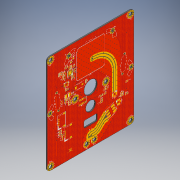
# Autodesk Inventor part: +XPanel_PCB
Saved by Autodesk Inventor 2018 (Build 220112000, 112)
## iProperties
Created: 2018-10-25
Part Number: +XPanel_PCB
Material: Epoxy Resin
Document SubType Name: Modeling
Designer: Bradley
Density: 1.14 g/cm^3
Appearance: Smooth - Dark Gray
Author: Bradley
Autodesk Inventor part; units mm, degrees
ref_plane "YZ Plane" through (0, 0, 0) normal (1, 0, 0) x (0, 1, 0)
ref_plane "XZ Plane" through (0, 0, 0) normal (0, 1, 0) x (-1, 0, 0)
ref_plane "XY Plane" through (0, 0, 0) normal (0, 0, 1) x (1, 0, 0)
sketch "Sketch1" plane through (0, 0, 0) normal (1, 0, 0) x (0, 1, 0)
  line L0 (36.5, -42) -> (-36.5, -42) construction
  line L1 (-36.5, -42) -> (-36.5, 42) construction
  line L2 (-36.5, 42) -> (36.5, 42) construction
  line L3 (36.5, 42) -> (36.5, -42) construction
  line L4 (36.5, -42) -> (-36.5, 42) construction
  line L5 (-36.5, -42) -> (36.5, 42) construction
  line L6 (-14, 0) -> (14, 0) construction
  line L7 (-39.5, -42) -> (-39.5, 42)
  arc A0 (-36.5, 45) -> (-39.5, 42) centre (-36.5, 42) ccw
  line L8 (-36.5, 45) -> (36.5, 45)
  arc A1 (39.5, 42) -> (36.5, 45) centre (36.5, 42) ccw
  line L9 (39.5, 42) -> (39.5, -42)
  arc A2 (36.5, -45) -> (39.5, -42) centre (36.5, -42) ccw
  line L10 (36.5, -45) -> (-36.5, -45)
  arc A3 (-39.5, -42) -> (-36.5, -45) centre (-36.5, -42) ccw
  point P0 (0, 0)
  point P1 (0, 0)
  dimension "d2" = 28
  dimension "d3" = 79
  dimension "d117" = 3
  dimension "d118" = 90
  dimension "d119" = 84
  dimension "d120" = 73
  constraints: 22 end point, 8 point on circle, 6 tangent, 4 centre point, 4 coincident, 4 midpoint, 4 parallel, 2 horizontal, 2 perpendicular, 1 equal radius, 1 vertical
  measures "d2" distance of L6.start L6.end
  measures "d3" distance between parallel lines of L9 L7
  measures "d117" radius of A0
  measures "d118" distance between parallel lines of L10 L8
  measures "d119" distance of L0.end L1.end
  measures "d120" distance of L1.end L2.end
extrude "Extrusion1" add sketch "Sketch1" along normal mid plane 1
sketch "Sketch3" plane through (0.5, 0, 0) normal (1, 0, 0) x (0, 0, -1)
  circle A0 centre (-2.5, 0) radius 6
  circle A1 centre (12.35, 0) radius 4.5
  line L0 (26, -6) -> (22, -6)
  line L1 (21, -5) -> (21, 5)
  line L2 (22, 6) -> (26, 6)
  line L3 (27, 5) -> (27, -5)
  line L4 (27, -6) -> (21, 6) construction
  line L5 (21, -6) -> (27, 6) construction
  arc A2 (21, -5) -> (22, -6) centre (22, -5) ccw
  arc A3 (26, -6) -> (27, -5) centre (26, -5) ccw
  arc A4 (27, 5) -> (26, 6) centre (26, 5) ccw
  arc A5 (22, 6) -> (21, 5) centre (22, 5) ccw
  point P0 (0, 0)
  point P1 (24, 0)
  point P2 (24, 0)
  dimension "d15" = 2.5
  dimension "d16" = 12
  dimension "d17" = 14.85
  dimension "d18" = 9
  dimension "d84" = 24
  dimension "d85" = 12
  dimension "d86" = 6
  dimension "d87" = 1
  constraints: 12 end point, 8 point on circle, 8 point on line, 8 tangent, 6 centre point, 3 equal radius, 3 horizontal alignment, 3 midpoint, 2 parallel, 1 horizontal, 1 perpendicular
  measures "d15" distance of point (0, 0) A0.centre
  measures "d16" diameter of A0
  measures "d17" distance of A1.centre A0.centre
  measures "d18" diameter of A1
  measures "d84" distance of point (0, 0) point (24, 0)
  measures "d85" distance of L5.start L4.end
  measures "d86" distance of L4.start L5.start
  measures "d87" radius of A2
extrude "Extrusion2" cut sketch "Sketch3" against normal through all
sketch "Sketch17" plane through (0.5, 0, 0) normal (1, 0, 0) x (0, 0, -1)
  line L0 (-45, 36.5) -> (-45, -36.5) projected
  line L1 (45, -36.5) -> (45, 36.5) projected
  line L2 (-45, -39.5061) -> (-45, 39.5061) construction
  line L3 (-45, 39.5061) -> (45, 39.5061) construction
  line L4 (45, 39.5061) -> (45, -39.5061) construction
  line L5 (45, -39.5061) -> (-45, -39.5061) construction
  point P0 (0, 0)
  point P1 (-45, 0)
  point P2 (-45, 0)
  constraints: 3 midpoint, 2 collinear, 2 other
decal "Decal4"
sketch "Sketch18" plane through (-0.5, 0, 0) normal (-1, 0, 0) x (0, 0, 1)
  line L0 (45, 39.5061) -> (45, -39.5061) construction
  line L1 (45, -39.5061) -> (-45, -39.5061) construction
  line L2 (-45, -39.5061) -> (-45, 39.5061) construction
  line L3 (-45, 39.5061) -> (45, 39.5061) construction
  line L4 (45, -36.5) -> (45, 36.5) projected
  line L5 (-45, 36.5) -> (-45, -36.5) projected
  point P0 (0, 0)
  point P1 (45, 0)
  constraints: 2 collinear, 2 midpoint, 2 other
decal "Decal5"
sketch "Sketch19" plane through (0.5, 0, 0) normal (1, 0, 0) x (0, 0, -1)
  point P0 (0, 0)
  point P1 (0, -14)
  point P2 (42, 36.5)
  point P3 (42, -36.5)
  point P4 (-42, -36.5)
  point P5 (0, 14)
  point P6 (-42, 36.5)
  constraints: 7 other
hole "Hole15" at (0.5, -14, 0) at (0.5, 36.5, -42) at (0.5, -36.5, -42) at (0.5, -36.5, 42) at (0.5, 14, 0) at (0.5, 36.5, 42) direction (-1, 0, 0) diameter 3.3 end through all
sketch "Sketch20" plane through (0.5, 0, 0) normal (1, 0, 0) x (0, 0, -1)
  point P0 (0, 0)
  point P1 (40.5, -3.5)
  point P2 (40.5, 3.5)
  constraints: 2 other
hole "Hole16" at (0.5, -3.5, -40.5) at (0.5, 3.5, -40.5) direction (-1, 0, 0) diameter 3 end through all
sketch "Sketch21" plane through (0.5, 0, 0) normal (1, 0, 0) x (0, 0, -1)
  point P0 (0, 0)
  point P1 (0, 37)
  point P2 (-37, 20)
  point P3 (0, -37)
  point P4 (-37, -20)
  constraints: 5 other
hole "Hole17" at (0.5, 37, 0) at (0.5, 20, 37) at (0.5, -37, 0) at (0.5, -20, 37) direction (-1, 0, 0) diameter 2.2 end through all
sketch "Sketch22" plane through (0.5, 0, 0) normal (1, 0, 0) x (0, 0, -1)
  point P0 (0, 0)
  point P1 (-13.444, 30.914)
  point P2 (1.444, -29.086)
  point P3 (-13.444, -30.914)
  point P4 (1.444, 29.086)
  constraints: 5 other
hole "Hole18" at (0.5, 30.914, 13.444) at (0.5, -29.086, -1.444) at (0.5, -30.914, 13.444) at (0.5, 29.086, -1.444) direction (-1, 0, 0) diameter 1 end through all
sketch "Sketch23" plane through (0.5, 0, 0) normal (1, 0, 0) x (0, 0, -1)
  point P0 (0, 0)
  point P1 (-24.25, 1.75)
  constraints: 1 other
hole "Hole19" at (0.5, 1.75, 24.25) direction (-1, 0, 0) diameter 0.95 end through all
sketch "Sketch24" plane through (0.5, 0, 0) normal (1, 0, 0) x (0, 0, -1)
  point P0 (0, 0)
  point P1 (36, 1)
  point P2 (36, -1)
  constraints: 2 other
hole "Hole20" at (0.5, 1, -36) at (0.5, -1, -36) direction (-1, 0, 0) diameter 0.7 end through all
sketch "Sketch25" plane through (0.5, 0, 0) normal (1, 0, 0) x (0, 0, -1)
  point P0 (0, 0)
  point P1 (-44.187, -37.211)
  point P2 (-44.187, -35.789)
  point P3 (-43.352, -34.639)
  point P4 (-42, -34.2)
  point P5 (43.352, -34.639)
  point P6 (44.187, -35.789)
  point P7 (44.187, -37.211)
  point P8 (43.352, -38.361)
  point P9 (42, -38.8)
  point P10 (40.648, -38.361)
  point P11 (39.813, -37.211)
  point P12 (39.813, -35.789)
  point P13 (40.648, -34.639)
  point P14 (42, -34.2)
  point P15 (2.187, -13.289)
  point P16 (2.187, -14.711)
  point P17 (1.352, -15.861)
  point P18 (0, -16.3)
  point P19 (-1.352, -15.861)
  point P20 (-2.187, -14.711)
  point P21 (-2.187, -13.289)
  point P22 (-1.352, -12.139)
  point P23 (0, -11.7)
  point P24 (38.4, -3.5)
  point P25 (39.015, -2.015)
  point P26 (40.5, -1.4)
  point P27 (41.985, 4.985)
  point P28 (42.6, 3.5)
  point P29 (41.985, 2.015)
  point P30 (40.5, 1.4)
  point P31 (39.015, 2.015)
  point P32 (38.4, 3.5)
  point P33 (39.015, 4.985)
  point P34 (40.5, 5.6)
  point P35 (1.352, -12.139)
  point P36 (-43.352, 38.361)
  point P37 (-42, 38.8)
  point P38 (-40.648, -34.639)
  point P39 (1.352, 15.861)
  point P40 (2.187, 14.711)
  point P41 (2.187, 13.289)
  point P42 (1.352, 12.139)
  point P43 (0, 11.7)
  point P44 (-1.352, 12.139)
  point P45 (-2.187, 13.289)
  point P46 (-2.187, 14.711)
  point P47 (-1.352, 15.861)
  point P48 (0, 16.3)
  point P49 (-39.813, -35.789)
  point P50 (43.352, 38.361)
  point P51 (44.187, 37.211)
  point P52 (44.187, 35.789)
  point P53 (43.352, 34.639)
  point P54 (42, 34.2)
  point P55 (40.648, 34.639)
  point P56 (39.813, 35.789)
  point P57 (39.813, 37.211)
  point P58 (40.648, 38.361)
  point P59 (42, 38.8)
  point P60 (-39.813, -37.211)
  point P61 (-40.648, 38.361)
  point P62 (-39.813, 37.211)
  point P63 (-39.813, 35.789)
  point P64 (-40.648, 34.639)
  point P65 (-42, 34.2)
  point P66 (-43.352, 34.639)
  point P67 (-44.187, 35.789)
  point P68 (39.015, -4.985)
  point P69 (40.5, -5.6)
  point P70 (41.985, -4.985)
  point P71 (42.6, -3.5)
  point P72 (41.985, -2.015)
  point P73 (-40.648, -38.361)
  point P74 (-42, -38.8)
  point P75 (-43.352, -38.361)
  point P76 (-44.187, 37.211)
  constraints: 56 other
hole "Hole21" at (0.5, -37.211, 44.187) at (0.5, -35.789, 44.187) at (0.5, -34.639, 43.352) at (0.5, -34.2, 42) at (0.5, -34.639, -43.352) at (0.5, -35.789, -44.187) at (0.5, -37.211, -44.187) at (0.5, -38.361, -43.352) at (0.5, -38.8, -42) at (0.5, -38.361, -40.648) at (0.5, -37.211, -39.813) at (0.5, -35.789, -39.813) at (0.5, -34.639, -40.648) at (0.5, -34.2, -42) at (0.5, -13.289, -2.187) at (0.5, -14.711, -2.187) at (0.5, -15.861, -1.352) at (0.5, -16.3, 0) at (0.5, -15.861, 1.352) at (0.5, -14.711, 2.187) at (0.5, -13.289, 2.187) at (0.5, -12.139, 1.352) at (0.5, -11.7, 0) at (0.5, -3.5, -38.4) at (0.5, -2.015, -39.015) at (0.5, -1.4, -40.5) at (0.5, 4.985, -41.985) at (0.5, 3.5, -42.6) at (0.5, 2.015, -41.985) at (0.5, 1.4, -40.5) at (0.5, 2.015, -39.015) at (0.5, 3.5, -38.4) at (0.5, 4.985, -39.015) at (0.5, 5.6, -40.5) at (0.5, -12.139, -1.352) at (0.5, 38.361, 43.352) at (0.5, 38.8, 42) at (0.5, -34.639, 40.648) at (0.5, 15.861, -1.352) at (0.5, 14.711, -2.187) at (0.5, 13.289, -2.187) at (0.5, 12.139, -1.352) at (0.5, 11.7, 0) at (0.5, 12.139, 1.352) at (0.5, 13.289, 2.187) at (0.5, 14.711, 2.187) at (0.5, 15.861, 1.352) at (0.5, 16.3, 0) at (0.5, -35.789, 39.813) at (0.5, 38.361, -43.352) direction (-1, 0, 0) diameter 0.45 end through all and at (0.5, 37.211, -44.187) (0.5, 35.789, -44.187) (0.5, 34.639, -43.352) (0.5, 34.2, -42) (0.5, 34.639, -40.648) (0.5, 35.789, -39.813) (0.5, 37.211, -39.813) (0.5, 38.361, -40.648) (0.5, 38.8, -42) (0.5, -37.211, 39.813) (0.5, 38.361, 40.648) (0.5, 37.211, 39.813) (0.5, 35.789, 39.813) (0.5, 34.639, 40.648) (0.5, 34.2, 42) (0.5, 34.639, 43.352) (0.5, 35.789, 44.187) (0.5, -4.985, -39.015) (0.5, -5.6, -40.5) (0.5, -4.985, -41.985) (0.5, -3.5, -42.6) (0.5, -2.015, -41.985) (0.5, -38.361, 40.648) (0.5, -38.8, 42) (0.5, -38.361, 43.352) (0.5, 37.211, 44.187)
sketch "Sketch26" plane through (0.5, 0, 0) normal (1, 0, 0) x (0, 0, -1)
  point P0 (0, 0)
  point P1 (-25.857, -13.857)
  point P2 (-7.735, -16.565)
  point P3 (-10, -19)
  point P4 (-3, -18)
  point P5 (-5, -18)
  point P6 (-10, -20)
  point P7 (-10, -22.095)
  point P8 (-27, -21)
  point P9 (-12, -12)
  point P10 (-5.627, -13.373)
  point P11 (8, 10)
  point P12 (-10, -1)
  point P13 (-7.15, -17.15)
  point P14 (-7, -15)
  point P15 (-27, -19.525)
  point P16 (-27, -23)
  point P17 (-4, -24)
  point P18 (-2.095, -20)
  point P19 (-30, -16.585)
  point P20 (-31, -15.415)
  point P21 (-17.75, -23)
  point P22 (-9, -22.095)
  point P23 (-10.585, -20.925)
  point P24 (-26, -21)
  point P25 (-19.95, -21.95)
  point P26 (-21.965, -23)
  point P27 (-25, -22)
  point P28 (-3, -17)
  point P29 (-5, -16)
  point P30 (-10, -16)
  point P31 (-9, -17)
  point P32 (-17.365, -15.585)
  point P33 (-17.574, -14.34)
  point P34 (8, -31)
  point P35 (23, -28)
  point P36 (3, -31)
  point P37 (3, -36)
  point P38 (-19, -27)
  point P39 (0, -22)
  point P40 (-20.17, -19.285)
  point P41 (-20.46, -16.916)
  point P42 (-14, -23.895)
  point P43 (-28, -16)
  point P44 (-16, -25.065)
  point P45 (6.775, -4)
  point P46 (4.955, -8)
  point P47 (6, -12)
  point P48 (-6, -26)
  point P49 (-11, -19)
  point P50 (-5.75, -24.75)
  point P51 (5, -3)
  point P52 (9, -5)
  point P53 (8, 6)
  point P54 (-14.167, -14.34)
  point P55 (7.585, 4)
  point P56 (3, 5.815)
  point P57 (-10, -11)
  point P58 (-10.085, -13.83)
  point P59 (-21.087, -15.888)
  point P60 (-3, -9)
  point P61 (-1, -9)
  point P62 (10, -7)
  point P63 (2, -9)
  point P64 (-28, -21)
  point P65 (0, -7.985)
  point P66 (-25, -15.085)
  point P67 (-23.1, -16)
  point P68 (6.775, 0)
  point P69 (2, -6)
  point P70 (-24, -15.965)
  point P71 (-21.733, -13.588)
  point P72 (-12.585, -10.93)
  point P73 (3, -5)
  point P74 (-21, -14)
  point P75 (-25, -16)
  point P76 (-24.346, -13.205)
  point P77 (24, 12)
  point P78 (22, 14)
  point P79 (20, 16)
  point P80 (20, 20)
  point P81 (26, 10)
  point P82 (28, 8)
  point P83 (30, 6)
  point P84 (32, 4)
  point P85 (32, 0)
  point P86 (30, 2)
  point P87 (28, 4)
  point P88 (28, 0)
  point P89 (30, -2)
  point P90 (32, -4)
  point P91 (34, -6)
  point P92 (38, -6)
  point P93 (36, -4)
  point P94 (34, -2)
  point P95 (20, 24)
  point P96 (20, 28)
  point P97 (23.9, 27.8)
  point P98 (26, 26)
  point P99 (28, 24)
  point P100 (30, 22)
  point P101 (24, 24)
  point P102 (28, 20)
  point P103 (32, 20)
  point P104 (34, 18)
  point P105 (36, 16)
  point P106 (38, 14)
  point P107 (40, 12)
  point P108 (42, 10)
  point P109 (40, 8)
  point P110 (38, 10)
  point P111 (36, 12)
  point P112 (34, 14)
  point P113 (32, 16)
  point P114 (32, 12)
  point P115 (34, 10)
  point P116 (36, 8)
  point P117 (38, 6)
  point P118 (-19.365, -22.535)
  point P119 (13, -34)
  point P120 (13, -31)
  point P121 (-18, -31)
  point P122 (-42, -19)
  point P123 (-16, -26)
  point P124 (22, -30)
  point P125 (24, -31)
  point P126 (18, -30)
  point P127 (17, 34)
  point P128 (15, 33)
  point P129 (-29, 33)
  point P130 (18, 25)
  point P131 (7, 14)
  point P132 (3.034, -11.034)
  point P133 (-27.25, -26)
  point P134 (-0.851, -24.149)
  point P135 (2.25, -17.5)
  point P136 (-12, -13)
  point P137 (-19, -19)
  point P138 (0, 38.6)
  point P139 (-1.131, 38.131)
  point P140 (-1.6, 37)
  point P141 (-1.131, 35.869)
  point P142 (0, 35.4)
  point P143 (1.131, 35.869)
  point P144 (1.6, 37)
  point P145 (1.131, 38.131)
  point P146 (-37, -18.4)
  point P147 (-38.131, -18.869)
  point P148 (-38.6, -20)
  point P149 (-38.131, -21.131)
  point P150 (-37, -21.6)
  point P151 (-35.869, -21.131)
  point P152 (-35.4, -20)
  point P153 (-35.869, -18.869)
  point P154 (0, -35.4)
  point P155 (-1.131, -35.869)
  point P156 (-1.6, -37)
  point P157 (-1.131, -38.131)
  point P158 (0, -38.6)
  point P159 (1.131, -38.131)
  point P160 (1.6, -37)
  point P161 (1.131, -35.869)
  point P162 (-37, 21.6)
  point P163 (-38.131, 21.131)
  point P164 (-38.6, 20)
  point P165 (-38.131, 18.869)
  point P166 (-37, 18.4)
  point P167 (-35.869, 18.869)
  point P168 (-35.4, 20)
  point P169 (-35.869, 21.131)
  point P170 (22, -24)
  point P171 (22, -26)
  point P172 (-8.085, -23)
  point P173 (-9, -15)
  point P174 (-3.02, -23.98)
  point P175 (-19.65, -16.9)
  point P176 (-26, -22)
  point P177 (-19.159, -19.841)
  point P178 (-23.243, -13.757)
  constraints: 179 other
hole "Hole22" at (0.5, -13.857, 25.857) at (0.5, -16.565, 7.735) at (0.5, -19, 10) at (0.5, -18, 3) at (0.5, -18, 5) at (0.5, -20, 10) at (0.5, -22.095, 10) at (0.5, -21, 27) at (0.5, -12, 12) at (0.5, -13.373, 5.627) at (0.5, 10, -8) at (0.5, -1, 10) at (0.5, -17.15, 7.15) at (0.5, -15, 7) at (0.5, -19.525, 27) at (0.5, -23, 27) at (0.5, -24, 4) at (0.5, -20, 2.095) at (0.5, -16.585, 30) at (0.5, -15.415, 31) at (0.5, -23, 17.75) at (0.5, -22.095, 9) at (0.5, -20.925, 10.585) at (0.5, -21, 26) at (0.5, -21.95, 19.95) at (0.5, -23, 21.965) at (0.5, -22, 25) at (0.5, -17, 3) at (0.5, -16, 5) at (0.5, -16, 10) at (0.5, -17, 9) at (0.5, -15.585, 17.365) at (0.5, -14.34, 17.574) at (0.5, -31, -8) at (0.5, -28, -23) at (0.5, -31, -3) at (0.5, -36, -3) at (0.5, -27, 19) at (0.5, -22, 0) at (0.5, -19.285, 20.17) at (0.5, -16.916, 20.46) at (0.5, -23.895, 14) at (0.5, -16, 28) at (0.5, -25.065, 16) at (0.5, -4, -6.775) at (0.5, -8, -4.955) at (0.5, -12, -6) at (0.5, -26, 6) at (0.5, -19, 11) at (0.5, -24.75, 5.75) direction (-1, 0, 0) diameter 0.35 end through all and at (0.5, -3, -5) (0.5, -5, -9) (0.5, 6, -8) (0.5, -14.34, 14.167) (0.5, 4, -7.585) (0.5, 5.815, -3) (0.5, -11, 10) (0.5, -13.83, 10.085) (0.5, -15.888, 21.087) (0.5, -9, 3) (0.5, -9, 1) (0.5, -7, -10) (0.5, -9, -2) (0.5, -21, 28) (0.5, -7.985, 0) (0.5, -15.085, 25) (0.5, -16, 23.1) (0.5, 0, -6.775) (0.5, -6, -2) (0.5, -15.965, 24) (0.5, -13.588, 21.733) (0.5, -10.93, 12.585) (0.5, -5, -3) (0.5, -14, 21) (0.5, -16, 25) (0.5, -13.205, 24.346) (0.5, 12, -24) (0.5, 14, -22) (0.5, 16, -20) (0.5, 20, -20) (0.5, 10, -26) (0.5, 8, -28) (0.5, 6, -30) (0.5, 4, -32) (0.5, 0, -32) (0.5, 2, -30) (0.5, 4, -28) (0.5, 0, -28) (0.5, -2, -30) (0.5, -4, -32) (0.5, -6, -34) (0.5, -6, -38) (0.5, -4, -36) (0.5, -2, -34) (0.5, 24, -20) (0.5, 28, -20) (0.5, 27.8, -23.9) (0.5, 26, -26) (0.5, 24, -28) (0.5, 22, -30) (0.5, 24, -24) (0.5, 20, -28) (0.5, 20, -32) (0.5, 18, -34) (0.5, 16, -36) (0.5, 14, -38) (0.5, 12, -40) (0.5, 10, -42) (0.5, 8, -40) (0.5, 10, -38) (0.5, 12, -36) (0.5, 14, -34) (0.5, 16, -32) (0.5, 12, -32) (0.5, 10, -34) (0.5, 8, -36) (0.5, 6, -38) (0.5, -22.535, 19.365) (0.5, -34, -13) (0.5, -31, -13) (0.5, -31, 18) (0.5, -19, 42) (0.5, -26, 16) (0.5, -30, -22) (0.5, -31, -24) (0.5, -30, -18) (0.5, 34, -17) (0.5, 33, -15) (0.5, 33, 29) (0.5, 25, -18) (0.5, 14, -7) (0.5, -11.034, -3.034) (0.5, -26, 27.25) (0.5, -24.149, 0.851) (0.5, -17.5, -2.25) (0.5, -13, 12) (0.5, -19, 19) (0.5, 38.6, 0) (0.5, 38.131, 1.131) (0.5, 37, 1.6) (0.5, 35.869, 1.131) (0.5, 35.4, 0) (0.5, 35.869, -1.131) (0.5, 37, -1.6) (0.5, 38.131, -1.131) (0.5, -18.4, 37) (0.5, -18.869, 38.131) (0.5, -20, 38.6) (0.5, -21.131, 38.131) (0.5, -21.6, 37) (0.5, -21.131, 35.869) (0.5, -20, 35.4) (0.5, -18.869, 35.869) (0.5, -35.4, 0) (0.5, -35.869, 1.131) (0.5, -37, 1.6) (0.5, -38.131, 1.131) (0.5, -38.6, 0) (0.5, -38.131, -1.131) (0.5, -37, -1.6) (0.5, -35.869, -1.131) (0.5, 21.6, 37) (0.5, 21.131, 38.131) (0.5, 20, 38.6) (0.5, 18.869, 38.131) (0.5, 18.4, 37) (0.5, 18.869, 35.869) (0.5, 20, 35.4) (0.5, 21.131, 35.869) (0.5, -24, -22) (0.5, -26, -22) (0.5, -23, 8.085) (0.5, -15, 9) (0.5, -23.98, 3.02) (0.5, -16.9, 19.65) (0.5, -22, 26) (0.5, -19.841, 19.159) (0.5, -13.757, 23.243)
sketch "Sketch27" plane through (0.5, 0, 0) normal (1, 0, 0) x (0, 0, -1)
  point P0 (0, 0)
  point P1 (-36, 16)
  point P2 (-32, 20)
  point P3 (-16, 16)
  point P4 (-18, 14)
  point P5 (-20, 12)
  point P6 (-18, -10)
  point P7 (-22, -10)
  point P8 (-16, -12)
  point P9 (-20, -12)
  point P10 (-24, -12)
  point P11 (-28, -12)
  point P12 (-32, -12)
  point P13 (-36, -12)
  point P14 (-26, -10)
  point P15 (-30, -10)
  point P16 (-34, -10)
  point P17 (-28, -8)
  point P18 (-32, -8)
  point P19 (-36, -8)
  point P20 (-26, -6)
  point P21 (-30, -6)
  point P22 (-34, -6)
  point P23 (-28, -4)
  point P24 (-32, -4)
  point P25 (-24, -8)
  point P26 (-20, -8)
  point P27 (-36, -4)
  point P28 (-26, -2)
  point P29 (-30, -2)
  point P30 (-34, -2)
  point P31 (-28, 0)
  point P32 (-32, 0)
  point P33 (-36, 0)
  point P34 (-26, 2)
  point P35 (-16, -8)
  point P36 (-22, -6)
  point P37 (-18, -6)
  point P38 (-14, -6)
  point P39 (-24, -4)
  point P40 (-20, -4)
  point P41 (-16, -4)
  point P42 (-22, -2)
  point P43 (-18, -2)
  point P44 (-14, -2)
  point P45 (-24, 0)
  point P46 (-20, 0)
  point P47 (-30, 2)
  point P48 (-34, 2)
  point P49 (-28, 4)
  point P50 (-32, 4)
  point P51 (-36, 4)
  point P52 (-26, 6)
  point P53 (-30, 6)
  point P54 (-34, 6)
  point P55 (-16, 0)
  point P56 (-28, 8)
  point P57 (-32, 8)
  point P58 (-36, 8)
  point P59 (-26, 10)
  point P60 (-30, 10)
  point P61 (-34, 10)
  point P62 (-24, 12)
  point P63 (-28, 12)
  point P64 (-22, 2)
  point P65 (-32, 12)
  point P66 (-26, 14)
  point P67 (-30, 14)
  point P68 (-34, 14)
  point P69 (-24, 16)
  point P70 (-28, 16)
  point P71 (-32, 16)
  point P72 (-26, 18)
  point P73 (-18, 2)
  point P74 (-14, 2)
  point P75 (-20, 4)
  point P76 (-16, 4)
  point P77 (-22, 6)
  point P78 (-18, 6)
  point P79 (-14, 6)
  point P80 (-20, 8)
  point P81 (-16, 8)
  point P82 (-12, 8)
  point P83 (-18, 10)
  point P84 (-14, 10)
  point P85 (-10, 10)
  point P86 (-16, 12)
  point P87 (-12, 12)
  point P88 (-8, 12)
  point P89 (-14, 14)
  point P90 (-10, 14)
  point P91 (-6, 14)
  point P92 (-12, 16)
  point P93 (-8, 16)
  point P94 (-4, 16)
  point P95 (-28, 20)
  point P96 (-28, 24)
  point P97 (-30, 22)
  point P98 (-14, -10)
  point P99 (-26, 22)
  point P100 (-22, 22)
  point P101 (-14, 22)
  point P102 (-18, 22)
  point P103 (-22, 18)
  point P104 (-14, 18)
  point P105 (-10, 18)
  point P106 (-6, 18)
  point P107 (-2, 18)
  point P108 (2, 18)
  point P109 (6, 18)
  point P110 (10, 18)
  point P111 (14, 18)
  point P112 (-24, 20)
  point P113 (-20, 20)
  point P114 (-8, 20)
  point P115 (-4, 20)
  point P116 (0, 20)
  point P117 (4, 20)
  point P118 (8, 20)
  point P119 (12, 20)
  point P120 (-24, 24)
  point P121 (-20, 24)
  point P122 (-16, 24)
  point P123 (-12, 24)
  point P124 (-8, 24)
  point P125 (-4, 24)
  point P126 (0, 24)
  point P127 (4, 24)
  point P128 (8, 24)
  point P129 (12, 24)
  point P130 (-22, 26)
  point P131 (-18, 26)
  point P132 (-14, 26)
  point P133 (-10, 26)
  point P134 (-6, 26)
  point P135 (-2, 26)
  point P136 (2, 26)
  point P137 (6, 26)
  point P138 (10, 26)
  point P139 (14, 26)
  point P140 (16, 24)
  point P141 (14, 22)
  point P142 (16, 20)
  point P143 (-30, 18)
  point P144 (-34, 18)
  point P145 (-38, -10)
  point P146 (-38, -6)
  point P147 (-38, -2)
  point P148 (-38, 2)
  point P149 (-38, 6)
  point P150 (-38, 10)
  point P151 (-36, 12)
  constraints: 152 other
hole "Hole23" at (0.5, 16, 36) at (0.5, 20, 32) at (0.5, 16, 16) at (0.5, 14, 18) at (0.5, 12, 20) at (0.5, -10, 18) at (0.5, -10, 22) at (0.5, -12, 16) at (0.5, -12, 20) at (0.5, -12, 24) at (0.5, -12, 28) at (0.5, -12, 32) at (0.5, -12, 36) at (0.5, -10, 26) at (0.5, -10, 30) at (0.5, -10, 34) at (0.5, -8, 28) at (0.5, -8, 32) at (0.5, -8, 36) at (0.5, -6, 26) at (0.5, -6, 30) at (0.5, -6, 34) at (0.5, -4, 28) at (0.5, -4, 32) at (0.5, -8, 24) at (0.5, -8, 20) at (0.5, -4, 36) at (0.5, -2, 26) at (0.5, -2, 30) at (0.5, -2, 34) at (0.5, 0, 28) at (0.5, 0, 32) at (0.5, 0, 36) at (0.5, 2, 26) at (0.5, -8, 16) at (0.5, -6, 22) at (0.5, -6, 18) at (0.5, -6, 14) at (0.5, -4, 24) at (0.5, -4, 20) at (0.5, -4, 16) at (0.5, -2, 22) at (0.5, -2, 18) at (0.5, -2, 14) at (0.5, 0, 24) at (0.5, 0, 20) at (0.5, 2, 30) at (0.5, 2, 34) at (0.5, 4, 28) at (0.5, 4, 32) direction (-1, 0, 0) diameter 0.3 end through all and at (0.5, 4, 36) (0.5, 6, 26) (0.5, 6, 30) (0.5, 6, 34) (0.5, 0, 16) (0.5, 8, 28) (0.5, 8, 32) (0.5, 8, 36) (0.5, 10, 26) (0.5, 10, 30) (0.5, 10, 34) (0.5, 12, 24) (0.5, 12, 28) (0.5, 2, 22) (0.5, 12, 32) (0.5, 14, 26) (0.5, 14, 30) (0.5, 14, 34) (0.5, 16, 24) (0.5, 16, 28) (0.5, 16, 32) (0.5, 18, 26) (0.5, 2, 18) (0.5, 2, 14) (0.5, 4, 20) (0.5, 4, 16) (0.5, 6, 22) (0.5, 6, 18) (0.5, 6, 14) (0.5, 8, 20) (0.5, 8, 16) (0.5, 8, 12) (0.5, 10, 18) (0.5, 10, 14) (0.5, 10, 10) (0.5, 12, 16) (0.5, 12, 12) (0.5, 12, 8) (0.5, 14, 14) (0.5, 14, 10) (0.5, 14, 6) (0.5, 16, 12) (0.5, 16, 8) (0.5, 16, 4) (0.5, 20, 28) (0.5, 24, 28) (0.5, 22, 30) (0.5, -10, 14) (0.5, 22, 26) (0.5, 22, 22) (0.5, 22, 14) (0.5, 22, 18) (0.5, 18, 22) (0.5, 18, 14) (0.5, 18, 10) (0.5, 18, 6) (0.5, 18, 2) (0.5, 18, -2) (0.5, 18, -6) (0.5, 18, -10) (0.5, 18, -14) (0.5, 20, 24) (0.5, 20, 20) (0.5, 20, 8) (0.5, 20, 4) (0.5, 20, 0) (0.5, 20, -4) (0.5, 20, -8) (0.5, 20, -12) (0.5, 24, 24) (0.5, 24, 20) (0.5, 24, 16) (0.5, 24, 12) (0.5, 24, 8) (0.5, 24, 4) (0.5, 24, 0) (0.5, 24, -4) (0.5, 24, -8) (0.5, 24, -12) (0.5, 26, 22) (0.5, 26, 18) (0.5, 26, 14) (0.5, 26, 10) (0.5, 26, 6) (0.5, 26, 2) (0.5, 26, -2) (0.5, 26, -6) (0.5, 26, -10) (0.5, 26, -14) (0.5, 24, -16) (0.5, 22, -14) (0.5, 20, -16) (0.5, 18, 30) (0.5, 18, 34) (0.5, -10, 38) (0.5, -6, 38) (0.5, -2, 38) (0.5, 2, 38) (0.5, 6, 38) (0.5, 10, 38) (0.5, 12, 36)
body "Solid1"
